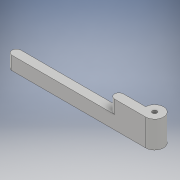
# Autodesk Inventor part: Traba
Saved by Autodesk Inventor 2017 (Build 210142000, 142)
## iProperties
Created: 2017-01-19
Part Number: Traba
Material: Generic
Document SubType Name: Modeling
Designer: A. Matías Quezada
Density: 1 g/cm^3
Appearance: Default
Author: A. Matías Quezada
Autodesk Inventor part; units mm, degrees
ref_plane "YZ Plane" through (0, 0, 0) normal (1, 0, 0) x (0, 1, 0)
ref_plane "XZ Plane" through (0, 0, 0) normal (0, 1, 0) x (-1, 0, 0)
ref_plane "XY Plane" through (0, 0, 0) normal (0, 0, 1) x (1, 0, 0)
sketch "Sketch1" plane through (0, 0, 0) normal (0, 0, 1) x (1, 0, 0)
  line L0 (0, 0) -> (-4, 0)
  line L1 (-4, 0) -> (-4, 4)
  line L2 (-4, 4) -> (0, 4)
  line L3 (0, 4) -> (0, 0)
  line L4 (-4, 0) -> (-33, 0)
  line L5 (-33, 0) -> (-33, 2)
  line L6 (-33, 2) -> (-4, 2)
  line L7 (-4, 2) -> (-4, 0)
  dimension "d1" = 4
  dimension "d3" = 29
  dimension "d4" = 2
  constraints: 16 end point, 4 parallel, 3 perpendicular, 2 horizontal
  measures "d1" distance of L1.end L2.end
  measures "d3" distance of L5.end L6.end
  measures "d4" distance of L4.end L5.end
extrude "Soporte Hoja" add sketch "Sketch1" along normal blind 3
fillet "Cabeza" radius 2 3 edges at (0, 0, 1.5) (0, 4, 1.5) (-4, 4, 1.5)
fillet "Agarre Hoja" radius 1 2 edges at (-33, 0, 1.5) (-33, 2, 1.5)
sketch "Sketch2" plane through (0, 0, 3) normal (0, 0, 1) x (1, 0, 0)
  circle A0 centre (-2, 2) radius 0.5
  arc A1 (-2, 0) -> (-4, 2) centre (-2, 2) ccw projected
  point P0 (0, 0)
  dimension "d9" = 1
  constraints: 1 centre point, 1 concentric
  measures "d9" diameter of A0
hole "Eje" at (-2, 2, 3) direction (0, 0, -1) diameter 1 end through all
sketch "Sketch3" plane through (0, 0, 3) normal (0, 0, 1) x (1, 0, 0)
  line L0 (-4, 2) -> (-32, 2) projected
  line L1 (-32, 0) -> (-2, 0) projected
  line L2 (-4, 2) -> (-32, 2) projected
  line L3 (-10, 2) -> (-10, 0)
  line L4 (-32, 0) -> (-2, 0) projected
  arc A0 (-2, 0) -> (-4, 2) centre (-2, 2) ccw projected
  circle A1 centre (-2, 2) radius 0.5 projected
  point P0 (0, 0)
  dimension "d17" = 10
  constraints: 2 end point, 2 point on line, 1 perpendicular
  measures "d17" distance from line of point (0, 0) L3
extrude "Soporte Deslizador" add sketch "Sketch3" along normal blind 3
fillet "Agarre Deslizador" radius 1 2 edges at (-10, 0, 4.5) (-10, 2, 4.5)
equation "\"d1\" = traba_cabeza_ancho"
equation "\"d3\" = traba_largo"
equation "\"d4\" = traba_hoja_ancho"
equation "\"d5\" = traba_hoja_grosor"
equation "\"d7\" = 0.5 * traba_cabeza_ancho"
equation "\"d8\" = 0.5 * traba_hoja_ancho"
equation "\"d10\" = traba_eje_diametro"
equation "\"d17\" = traba_deslizador_largo"
equation "\"d18\" = traba_deslizador_alto"
equation "\"d20\" = 0.5 * traba_hoja_ancho"
equation "\"traba_cabeza_ancho\" = 4"
equation "\"traba_largo\" = 29"
equation "\"traba_hoja_ancho\" = 2"
equation "\"traba_hoja_grosor\" = 3"
equation "\"traba_eje_diametro\" = 1"
equation "\"traba_deslizador_alto\" = 3"
equation "\"traba_deslizador_largo\" = 10"
body "Solid1"
